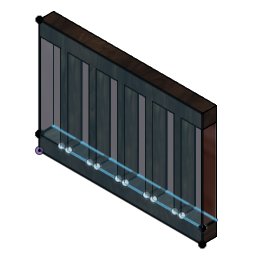
LED Fixture v4 (Autodesk Fusion 360 design; units mm, degrees)
Autodesk Fusion 360 part; units mm, degrees
note: some values were not read from the file. Chosen so that the rebuilt part matches the saved one: which bodies a step acts on.
sketch "Sketch2" plane through (0, 0, 0) normal (0, 1, 0) x (1, 0, 0)
sketch "Sketch3" plane through (0, 0, 0) normal (0, 1, 0) x (1, 0, 0)
  line L0 (0, 0) -> (584.2, 0)
  line L1 (584.2, 0) -> (584.2, -50.8)
  line L2 (584.2, -50.8) -> (0, -50.8)
  line L3 (0, -50.8) -> (0, 0)
  dimension "d1" = 584.2
  dimension "d2" = 50.8
  constraint horizontal L0
  constraint vertical L1
  constraint horizontal L2
  constraint vertical L3
  constraint coincident L0.start L3.end
  measures "d1" distance of L0.start L0.end
  measures "d2" distance of L0.start L2.end
extrude "Extrude1" add sketch "Sketch3" along normal blind 50.8 makes body 1
sketch "Sketch4" plane through (0, 0, 50.8) normal (0, 0, 1) x (-1, 0, 0)
  line L0 (0, 0) -> (-584.2, 0)
  line L1 (-584.2, 0) -> (-584.2, -50.8)
  line L2 (-584.2, -50.8) -> (0, -50.8)
  line L3 (0, -50.8) -> (0, 0)
  line L4 (0, 0) -> (-76.2, 0)
  line L5 (-76.2, 0) -> (-76.2, -50.8)
  line L6 (-76.2, -50.8) -> (0, -50.8)
  line L7 (0, -50.8) -> (0, 0)
  line L8 (-76.2, -50.8) -> (-101.6, -50.8)
  line L9 (-101.6, -50.8) -> (-101.6, 0)
  line L10 (-101.6, 0) -> (-76.2, 0)
  line L11 (-76.2, 0) -> (-76.2, -50.8)
  line L12 (-101.6, -50.8) -> (-177.8, -50.8)
  line L13 (-177.8, -50.8) -> (-177.8, 0)
  line L14 (-177.8, 0) -> (-101.6, 0)
  line L15 (-101.6, 0) -> (-101.6, -50.8)
  line L16 (-177.8, -50.8) -> (-203.2, -50.8)
  line L17 (-203.2, -50.8) -> (-203.2, 0)
  line L18 (-203.2, 0) -> (-177.8, 0)
  line L19 (-177.8, 0) -> (-177.8, -50.8)
  line L20 (-203.2, -50.8) -> (-279.4, -50.8)
  line L21 (-279.4, -50.8) -> (-279.4, 0)
  line L22 (-279.4, 0) -> (-203.2, 0)
  line L23 (-203.2, 0) -> (-203.2, -50.8)
  line L24 (-279.4, -50.8) -> (-304.8, -50.8)
  line L25 (-304.8, -50.8) -> (-304.8, 0)
  line L26 (-304.8, 0) -> (-279.4, 0)
  line L27 (-279.4, 0) -> (-279.4, -50.8)
  line L28 (-304.8, -50.8) -> (-381, -50.8)
  line L29 (-381, -50.8) -> (-381, 0)
  line L30 (-381, 0) -> (-304.8, 0)
  line L31 (-304.8, 0) -> (-304.8, -50.8)
  line L32 (-381, -50.8) -> (-406.4, -50.8)
  line L33 (-406.4, -50.8) -> (-406.4, 0)
  line L34 (-406.4, 0) -> (-381, 0)
  line L35 (-381, 0) -> (-381, -50.8)
  line L36 (-406.4, -50.8) -> (-482.6, -50.8)
  line L37 (-482.6, -50.8) -> (-482.6, 0)
  line L38 (-482.6, 0) -> (-406.4, 0)
  line L39 (-406.4, 0) -> (-406.4, -50.8)
  line L40 (-482.6, -50.8) -> (-508, -50.8)
  line L41 (-508, -50.8) -> (-508, 0)
  line L42 (-508, 0) -> (-482.6, 0)
  line L43 (-482.6, 0) -> (-482.6, -50.8)
  line L44 (-508, -50.8) -> (-584.2, -50.8)
  line L45 (-584.2, -50.8) -> (-584.2, 0)
  line L46 (-584.2, 0) -> (-508, 0)
  line L47 (-508, 0) -> (-508, -50.8)
  line L48 (0, -50.8) -> (-3, -50.8)
  line L49 (-3, -50.8) -> (-3, 0)
  line L50 (-3, 0) -> (0, 0)
  line L51 (0, 0) -> (0, -50.8)
  line L52 (0, 0) -> (-76.2, 0)
  line L53 (-76.2, 0) -> (-76.2, -3)
  line L54 (0, -3) -> (0, 0)
  line L55 (-101.6, 0) -> (-177.8, 0)
  line L56 (-177.8, 0) -> (-177.8, -3)
  line L57 (-101.6, -3) -> (-101.6, 0)
  line L58 (-203.2, 0) -> (-279.4, 0)
  line L59 (-279.4, 0) -> (-279.4, -3)
  line L60 (-203.2, -3) -> (-203.2, 0)
  line L61 (-304.8, 0) -> (-381, 0)
  line L62 (-381, 0) -> (-381, -3)
  line L63 (-304.8, -3) -> (-304.8, 0)
  line L64 (-406.4, 0) -> (-482.6, 0)
  line L65 (-482.6, 0) -> (-482.6, -3)
  line L66 (-406.4, -3) -> (-406.4, 0)
  line L67 (-508, 0) -> (-584.2, 0)
  line L68 (-584.2, 0) -> (-584.2, -3)
  line L69 (-508, -3) -> (-508, 0)
  line L70 (-584.2, 0) -> (-581.2, 0)
  line L71 (-581.2, 0) -> (-581.2, -50.8)
  line L72 (-581.2, -50.8) -> (-584.2, -50.8)
  line L73 (-584.2, -50.8) -> (-584.2, 0)
  line L74 (-584.2, -50.8) -> (-508, -50.8)
  line L75 (-508, -50.8) -> (-508, -47.8)
  line L76 (-508, -47.8) -> (-584.2, -47.8)
  line L77 (-584.2, -47.8) -> (-584.2, -50.8)
  line L78 (-482.6, -50.8) -> (-406.4, -50.8)
  line L79 (-406.4, -50.8) -> (-406.4, -47.8)
  line L80 (-406.4, -47.8) -> (-482.6, -47.8)
  line L81 (-482.6, -47.8) -> (-482.6, -50.8)
  line L82 (-381, -50.8) -> (-304.8, -50.8)
  line L83 (-304.8, -50.8) -> (-304.8, -47.8)
  line L84 (-304.8, -47.8) -> (-381, -47.8)
  line L85 (-381, -47.8) -> (-381, -50.8)
  line L86 (-279.4, -50.8) -> (-203.2, -50.8)
  line L87 (-203.2, -50.8) -> (-203.2, -47.8)
  line L88 (-203.2, -47.8) -> (-279.4, -47.8)
  line L89 (-279.4, -47.8) -> (-279.4, -50.8)
  line L90 (-177.8, -50.8) -> (-101.6, -50.8)
  line L91 (-101.6, -50.8) -> (-101.6, -47.8)
  line L92 (-101.6, -47.8) -> (-177.8, -47.8)
  line L93 (-177.8, -47.8) -> (-177.8, -50.8)
  line L94 (-76.2, -50.8) -> (0, -50.8)
  line L95 (0, -50.8) -> (0, -47.8)
  line L96 (0, -47.8) -> (-76.2, -47.8)
  line L97 (-76.2, -47.8) -> (-76.2, -50.8)
  dimension "d5" = 76.2
  dimension "d6" = 25.4
  dimension "d7" = 76.2
  dimension "d8" = 25.4
  dimension "d9" = 76.2
  dimension "d10" = 25.4
  dimension "d11" = 76.2
  dimension "d12" = 25.4
  dimension "d13" = 76.2
  dimension "d14" = 25.4
  dimension "d15" = 76.2
  dimension "d24" = 3
  dimension "d25" = 3
  dimension "d26" = 3
  dimension "d27" = 3
  dimension "d28" = 3
  dimension "d29" = 3
  dimension "d30" = 3
  dimension "d31" = 3
  dimension "d32" = 3
  dimension "d33" = 3
  dimension "d34" = 3
  dimension "d35" = 3
  dimension "d36" = 3
  dimension "d37" = 3
  constraint horizontal L4
  constraint vertical L5
  constraint horizontal L6
  constraint vertical L7
  constraint coincident L0.start L3.end
  constraint horizontal L8
  constraint vertical L9
  constraint horizontal L10
  constraint vertical L11
  constraint horizontal L12
  constraint vertical L13
  constraint horizontal L14
  constraint vertical L15
  constraint horizontal L16
  constraint vertical L17
  constraint horizontal L18
  constraint vertical L19
  constraint horizontal L20
  constraint vertical L21
  constraint horizontal L22
  constraint vertical L23
  constraint horizontal L24
  constraint vertical L25
  constraint horizontal L26
  constraint vertical L27
  constraint horizontal L28
  constraint vertical L29
  constraint horizontal L30
  constraint vertical L31
  constraint horizontal L32
  constraint vertical L33
  constraint horizontal L34
  constraint vertical L35
  constraint horizontal L36
  constraint vertical L37
  constraint horizontal L38
  constraint vertical L39
  constraint horizontal L40
  constraint vertical L41
  constraint horizontal L42
  constraint vertical L43
  constraint horizontal L44
  constraint vertical L45
  constraint horizontal L46
  constraint vertical L47
  constraint horizontal L48
  constraint vertical L49
  constraint horizontal L50
  constraint vertical L51
  constraint horizontal L52
  constraint vertical L53
  constraint vertical L54
  constraint horizontal L55
  constraint vertical L56
  constraint vertical L57
  constraint horizontal L58
  constraint vertical L59
  constraint vertical L60
  constraint horizontal L61
  constraint vertical L62
  constraint vertical L63
  constraint horizontal L64
  constraint vertical L65
  constraint vertical L66
  constraint horizontal L67
  constraint vertical L68
  constraint vertical L69
  constraint horizontal L70
  constraint vertical L71
  constraint horizontal L72
  constraint vertical L73
  constraint coincident L0.end L1.start
  constraint horizontal L74
  constraint vertical L75
  constraint horizontal L76
  constraint vertical L77
  constraint coincident L47 L75.end
  constraint horizontal L78
  constraint vertical L79
  constraint horizontal L80
  constraint vertical L81
  constraint horizontal L82
  constraint vertical L83
  constraint horizontal L84
  constraint vertical L85
  constraint horizontal L86
  constraint vertical L87
  constraint horizontal L88
  constraint vertical L89
  constraint horizontal L90
  constraint vertical L91
  constraint horizontal L92
  constraint vertical L93
  constraint horizontal L94
  constraint vertical L95
  constraint horizontal L96
  constraint vertical L97
  measures "d5" distance of L0.start L4.end
  measures "d6" distance of L5.end L8.end
  measures "d7" distance of L8.end L12.end
  measures "d8" distance of L12.end L16.end
  measures "d9" distance of L16.end L20.end
  measures "d10" distance of L20.end L24.end
  measures "d11" distance of L24.end L28.end
  measures "d12" distance of L28.end L32.end
  measures "d13" distance of L32.end L36.end
  measures "d14" distance of L36.end L40.end
  measures "d15" distance of L40.end L1.end
  measures "d24" distance of L2.end L48.end
  measures "d25" distance of L0.start L54.start
  measures "d26" distance of L9.end L57.start
  measures "d27" distance of L17.end L60.start
  measures "d28" distance of L25.end L63.start
  measures "d29" distance of L33.end L66.start
  measures "d30" distance of L41.end L69.start
  measures "d31" distance of L0.end L70.end
  measures "d32" distance of L1.end L76.end
  measures "d33" distance of L36.end L80.end
  measures "d34" distance of L28.end L84.end
  measures "d35" distance of L20.end L88.end
  measures "d36" distance of L12.end L92.end
  measures "d37" distance of L5.end L96.end
sketch "Sketch5" plane through (0, 0, 0) normal (0, 1, 0) x (1, 0, 0)
extrude "Extrude2" add sketch "Sketch4" along normal blind 355.6 bodies 1
sketch "Sketch6" plane through (0, 0, 0) normal (0, -1, 0) x (1, 0, 0)
  line L0 (0, 406.4) -> (0, 0)
  line L1 (0, 0) -> (584.2, 0)
  line L2 (584.2, 0) -> (584.2, 406.4)
  line L3 (584.2, 406.4) -> (0, 406.4)
  line L4 (0, 0) -> (0, 50.8) construction
  line L5 (0, 50.8) -> (584.2, 50.8)
  line L6 (584.2, 50.8) -> (584.2, 355.6)
  line L7 (584.2, 355.6) -> (0, 355.6)
  line L8 (0, 355.6) -> (0, 50.8)
  dimension "d18" = 50.8
  dimension "d19" = 304.8
  constraint coincident L0.end L1.start
  constraint perpendicular L1 L4
  constraint horizontal L5
  constraint vertical L6
  constraint horizontal L7
  constraint vertical L8
  measures "d18" distance of L0.end L4.end
  measures "d19" distance of L4.end L7.end
extrude "Extrude3" cut sketch "Sketch6" against normal blind 325 contours L0 L2 L5 L6 L7 L8 bodies 1 makes body 2 at (194.7333, 0, 16.9333)
extrude "Extrude4" add sketch "Sketch4" along normal blind 304.8 contours L0 L2 L5 L8 L9 L10 L11 L15 L53 L57 L91 L97 | L0 L2 L13 L16 L17 L18 L19 L23 L56 L60 L87 L93 | L0 L2 L21 L24 L25 L26 L27 L31 L59 L63 L83 L89 | L0 L2 L29 L32 L33 L34 L35 L39 L62 L66 L79 L85 | L0 L2 L37 L40 L41 L42 L43 L47 L65 L69 L75 L81 bodies 1 2
extrude "Extrude5" add sketch "Sketch4" along normal blind 304.8 separate body contours L0 L3 L4 L7 L49 L50 L51 L52 L54 L96 | L2 L3 L6 L7 L48 L49 L51 L94 L95 L96 | L2 L5 L6 L11 L49 L94 L96 L97 | L2 L9 L12 L13 L15 L19 L90 L91 L92 L93 | L2 L17 L20 L21 L23 L27 L86 L87 L88 L89 | L2 L25 L28 L29 L31 L35 L82 L83 L84 L85 | L2 L33 L36 L37 L39 L43 L78 L79 L80 L81 | L0 L1 L45 L46 L67 L68 L70 L71 L73 L76 | L2 L41 L44 L47 L71 L74 L75 L76 | L1 L2 L44 L45 L71 L72 L73 L74 L76 L77 makes body 3 at (254, 50.8, 254) makes body 4 at (558.8, 50.8, 254) makes body 5 at (127, 47.8, 254) makes body 6 at (355.6, 50.8, 254) makes body 7 at (431.8, 47.8, 254) makes body 8 at (50.8, 50.8, 254)
sketch "Sketch7" plane through (0, 0, 0) normal (0, -1, 0) x (1, 0, 0)
  line L0 (482.6, 50.8) -> (406.4, 50.8)
  line L1 (406.4, 50.8) -> (406.4, 355.6)
  line L2 (406.4, 355.6) -> (482.6, 355.6)
  line L3 (482.6, 355.6) -> (482.6, 50.8)
  line L4 (508, 50.8) -> (508, 355.6)
  line L5 (508, 355.6) -> (584.2, 355.6)
  line L6 (584.2, 355.6) -> (584.2, 406.4)
  line L7 (584.2, 406.4) -> (0, 406.4)
  line L8 (0, 406.4) -> (0, 355.6)
  line L9 (0, 355.6) -> (76.2, 355.6)
  line L10 (76.2, 355.6) -> (76.2, 50.8)
  line L11 (76.2, 50.8) -> (0, 50.8)
  line L12 (0, 50.8) -> (0, 0)
  line L13 (0, 0) -> (584.2, 0)
  line L14 (584.2, 0) -> (584.2, 50.8)
  line L15 (584.2, 50.8) -> (508, 50.8)
  line L16 (381, 50.8) -> (304.8, 50.8)
  line L17 (304.8, 50.8) -> (304.8, 355.6)
  line L18 (304.8, 355.6) -> (381, 355.6)
  line L19 (381, 355.6) -> (381, 50.8)
  line L20 (101.6, 50.8) -> (101.6, 355.6)
  line L21 (101.6, 355.6) -> (177.8, 355.6)
  line L22 (177.8, 355.6) -> (177.8, 50.8)
  line L23 (177.8, 50.8) -> (101.6, 50.8)
  line L24 (203.2, 50.8) -> (203.2, 355.6)
  line L25 (203.2, 355.6) -> (279.4, 355.6)
  line L26 (279.4, 355.6) -> (279.4, 50.8)
  line L27 (279.4, 50.8) -> (203.2, 50.8)
  line L28 (0, 406.4) -> (584.2, 406.4)
  line L29 (584.2, 406.4) -> (584.2, 0)
  line L30 (584.2, 0) -> (0, 0)
  line L31 (0, 0) -> (0, 406.4)
  constraint horizontal L28
  constraint vertical L29
  constraint horizontal L30
  constraint vertical L31
  constraint coincident L13.end L14.start
  constraint coincident L7.end L8.start
sketch "Sketch8" plane through (292.1, 0, 203.2) normal (0, -1, 0) x (1, 0, 0)
sketch "Sketch9" plane through (0, 0, 0) normal (0, -1, 0) x (1, 0, 0)
  line L0 (0, 0) -> (584.2, 0)
  line L1 (584.2, 0) -> (584.2, 406.4)
  line L2 (584.2, 406.4) -> (0, 406.4)
  line L3 (0, 406.4) -> (0, 0)
  dimension "d40" = 584.2
  dimension "d41" = 406.4
  constraint horizontal L0
  constraint vertical L1
  constraint horizontal L2
  constraint vertical L3
  constraint coincident L0.start L3.end
  measures "d40" distance of L0.start L0.end
  measures "d41" distance of L0.start L2.end
